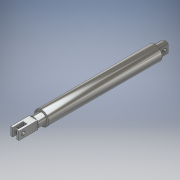
# Autodesk Inventor part: 4in stroke cylinder
Saved by Autodesk Inventor 2017 (Build 210142000, 142)
## iProperties
Created: 2017-01-19
Part Number: 4in stroke cylinder
Material: Generic
Document SubType Name: Modeling
Designer: Ben
Density: 1 g/cm^3
Appearance: Chrome - Polished
Author: Ben
Autodesk Inventor part; units mm, degrees
ref_plane "YZ Plane" through (0, 0, 0) normal (1, 0, 0) x (0, 1, 0)
ref_plane "XZ Plane" through (0, 0, 0) normal (0, 1, 0) x (-1, 0, 0)
ref_plane "XY Plane" through (0, 0, 0) normal (0, 0, 1) x (1, 0, 0)
sketch "Sketch1" plane through (0, 0, 0) normal (0, 0, 1) x (1, 0, 0)
  circle A0 centre (0, 0) radius 7.9375
  dimension "d0" = 15.875
  constraints: 1 centre point, 1 coincident
  measures "d0" diameter of A0
extrude "Extrusion1" add sketch "Sketch1" along normal blind 15.875
sketch "Sketch2" plane through (0, 0, 15.875) normal (0, 0, 1) x (1, 0, 0)
  circle A0 centre (0, 0) radius 11.1125
  dimension "d3" = 22.225
  constraints: 1 centre point, 1 coincident
  measures "d3" diameter of A0
extrude "Extrusion2" add sketch "Sketch2" along normal blind 174.625
sketch "Sketch3" plane through (0, 0, 190.5) normal (0, 0, 1) x (1, 0, 0)
  circle A0 centre (0, 0) radius 7.9375 projected
extrude "Extrusion3" add sketch "Sketch3" along normal blind 12.7
sketch "Sketch4" plane through (0, 0, 0) normal (0, 0, -1) x (-1, 0, 0)
  line L0 (-4.7625, 0) -> (4.7625, 0) construction
  line L1 (-4.7625, 14.2513) -> (-13.4248, 14.2513)
  line L2 (-13.4248, 14.2513) -> (-13.4248, -14.2513)
  line L3 (-13.4248, -14.2513) -> (-4.7625, -14.2513)
  line L4 (-4.7625, -14.2513) -> (-4.7625, 14.2513)
  line L5 (4.7625, 14.2513) -> (11.8991, 14.2513)
  line L6 (11.8991, 14.2513) -> (11.8991, -14.2513)
  line L7 (11.8991, -14.2513) -> (4.7625, -14.2513)
  line L8 (4.7625, -14.2513) -> (4.7625, 14.2513)
  point P0 (0, 0)
  point P1 (0, 0)
  dimension "d8" = 9.525
  constraints: 18 end point, 4 parallel, 3 horizontal, 3 midpoint, 2 perpendicular, 1 coincident, 1 point on line
  measures "d8" distance of L0.end L0.start
extrude "Extrusion4" cut sketch "Sketch4" against normal up to surface (15.875 mm away)
sketch "Sketch5" plane through (4.7625, -6.35, 0) normal (1, 0, 0) x (0, 0, -1)
  line L0 (0, 6.35) -> (-6.35, 6.35) construction
  circle A0 centre (-6.35, 6.35) radius 3.175
  dimension "d11" = 6.35
  dimension "d12" = 6.35
  constraints: 2 end point, 1 centre point, 1 coincident, 1 horizontal
  measures "d11" distance of L0.start L0.end
  measures "d12" diameter of A0
extrude "Extrusion5" cut sketch "Sketch5" against normal through all
sketch "Sketch6" plane through (0, 0, 203.2) normal (0, 0, 1) x (1, 0, 0)
  line L0 (-6.35, 6.35) -> (6.35, 6.35)
  line L1 (6.35, 6.35) -> (6.35, -6.35)
  line L2 (6.35, -6.35) -> (-6.35, -6.35)
  line L3 (-6.35, -6.35) -> (-6.35, 6.35)
  line L4 (0, 0) -> (0, 6.35) construction
  line L5 (0, 0) -> (-6.35, 0) construction
  dimension "d15" = 12.7
  constraints: 12 end point, 2 horizontal, 2 midpoint, 2 parallel, 2 perpendicular, 1 vertical
  measures "d15" distance of L0.start L0.end
extrude "Extrusion6" add sketch "Sketch6" along normal blind 28.575
sketch "Sketch7" plane through (0, 0, 231.775) normal (0, 0, 1) x (1, 0, 0)
  line L0 (-4.7625, 6.35) -> (4.7625, 6.35) projected
  line L1 (4.7625, -6.35) -> (-4.7625, -6.35) projected
  line L2 (-3.175, 6.35) -> (3.175, 6.35)
  line L3 (3.175, 6.35) -> (3.175, -6.35)
  line L4 (3.175, -6.35) -> (-3.175, -6.35)
  line L5 (-3.175, -6.35) -> (-3.175, 6.35)
  line L6 (-3.175, 0) -> (3.175, 0) construction
  point P0 (0, 0)
  point P1 (0, 0)
  dimension "d18" = 6.35
  constraints: 10 end point, 3 midpoint, 2 parallel, 2 point on line, 1 coincident, 1 horizontal, 1 perpendicular
  measures "d18" distance between parallel lines of L5 L3
extrude "Extrusion7" cut sketch "Sketch7" against normal blind 15.875
sketch "Sketch8" plane through (6.35, 4.7625, 203.2) normal (1, 0, 0) x (0, 0, -1)
  line L0 (-28.575, -11.1125) -> (-28.575, 1.5875) construction
  line L1 (-28.575, -4.7625) -> (-22.225, -4.7625) construction
  circle A0 centre (-22.225, -4.7625) radius 3.175
  point P0 (203.2, -4.7625)
  dimension "d21" = 6.35
  dimension "d22" = 6.35
  constraints: 2 end point, 1 centre point, 1 coincident, 1 horizontal, 1 midpoint
  measures "d21" distance of L1.start L1.end
  measures "d22" diameter of A0
extrude "Extrusion8" cut sketch "Sketch8" against normal through all
body "Solid1"
